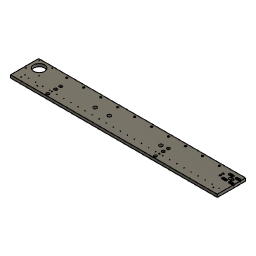
XPlate v29 (Autodesk Fusion 360 archive; units mm, degrees)
design "XPlate" references "tormach 770mx"
Autodesk Fusion 360 part; units mm, degrees
sketch "Sketch1" plane through (0, 0, 0) normal (0, 1, 0) x (1, 0, 0)
  line L0 (0, 0) -> (732, 0)
  line L1 (732, 0) -> (732, -100)
  line L2 (732, -100) -> (0, -100)
  line L3 (0, -100) -> (0, 0)
  dimension "d1" = 732
  dimension "d2" = 100
  constraint horizontal L0
  constraint vertical L1
  constraint horizontal L2
  constraint vertical L3
  constraint coincident L0.start L3.end
  measures "d1" distance of L0.start L0.end
  measures "d2" distance of L0.start L2.end
extrude "Extrude1" add sketch "Sketch1" along normal blind 9.6
sketch "Sketch2" plane through (0, 9.6, 0) normal (0, 1, 0) x (-1, 0, 0)
  line L0 (0, 100) -> (-732, 100)
  line L1 (-732, 100) -> (-732, 0)
  line L2 (-732, 0) -> (0, 0)
  line L3 (0, 0) -> (0, 100)
  line L4 (0, 28.5) -> (-732, 28.5) construction
  line L5 (-707, 23.5) -> (-713, 23.5)
  line L6 (-707, 33.5) -> (-712.9996, 33.5)
  arc A0 (-707, 23.5) -> (-707, 33.5) centre (-707, 28.5) ccw
  arc A1 (-712.9996, 33.5) -> (-713, 23.5) centre (-713, 28.5) ccw
  line L7 (0, 16.5) -> (-732, 16.5) construction
  line L8 (-693, 20.5) -> (-703, 20.5)
  arc A2 (-703, 20.5) -> (-703, 12.5) centre (-703, 16.5) ccw
  line L9 (-703, 12.5) -> (-693, 12.5)
  arc A3 (-693, 12.5) -> (-693, 20.5) centre (-693, 16.5) ccw
  line L10 (-693, 16.5) -> (-703, 16.5) construction
  line L11 (-717, 20.5) -> (-727, 20.5)
  arc A4 (-727, 20.5) -> (-727, 12.5) centre (-727, 16.5) ccw
  line L12 (-727, 12.5) -> (-717, 12.5)
  arc A5 (-717, 12.5) -> (-717, 20.5) centre (-717, 16.5) ccw
  line L13 (-717, 16.5) -> (-727, 16.5) construction
  line L14 (-694.5, 18.75) -> (-701.5, 18.75)
  arc A6 (-701.5, 18.75) -> (-701.5, 14.25) centre (-701.5, 16.5) ccw
  line L15 (-701.5, 14.25) -> (-694.5, 14.25)
  arc A7 (-694.5, 14.25) -> (-694.5, 18.75) centre (-694.5, 16.5) ccw
  line L16 (-694.5, 16.5) -> (-701.5, 16.5) construction
  line L17 (-718.5, 18.75) -> (-725.5, 18.75)
  arc A8 (-725.5, 18.75) -> (-725.5, 14.25) centre (-725.5, 16.5) ccw
  line L18 (-725.5, 14.25) -> (-718.5, 14.25)
  arc A9 (-718.5, 14.25) -> (-718.5, 18.75) centre (-718.5, 16.5) ccw
  line L19 (-718.5, 16.5) -> (-725.5, 16.5) construction
  line L20 (-693, 16.5) -> (-693, 44) construction
  line L21 (-694.5, 16.5) -> (-694.5, 18.75) construction
  line L22 (-703, 16.5) -> (-703, 44) construction
  line L23 (-694.5, 16.5) -> (-694.5, 44) construction
  line L24 (-701.5, 16.5) -> (-701.5, 44) construction
  line L25 (-717, 16.5) -> (-717, 44) construction
  line L26 (-718.5, 16.5) -> (-718.5, 44) construction
  line L27 (-725.5, 16.5) -> (-725.5, 44) construction
  line L28 (-727, 16.5) -> (-727, 44) construction
  line L29 (-689, 40.5) -> (-732, 40.5) construction
  line L30 (-694.5, 42.75) -> (-701.5, 42.75)
  arc A10 (-701.5, 42.75) -> (-701.5, 38.25) centre (-701.5, 40.5) ccw
  line L31 (-701.5, 38.25) -> (-694.5, 38.25)
  arc A11 (-694.5, 38.25) -> (-694.5, 42.75) centre (-694.5, 40.5) ccw
  line L32 (-694.5, 40.5) -> (-701.5, 40.5) construction
  line L33 (-693, 44.5) -> (-703, 44.5)
  arc A12 (-703, 44.5) -> (-703, 36.5) centre (-703, 40.5) ccw
  line L34 (-703, 36.5) -> (-693, 36.5)
  arc A13 (-693, 36.5) -> (-693, 44.5) centre (-693, 40.5) ccw
  line L35 (-693, 40.5) -> (-703, 40.5) construction
  line L36 (-718.5, 42.75) -> (-725.5, 42.75)
  arc A14 (-725.5, 42.75) -> (-725.5, 38.25) centre (-725.5, 40.5) ccw
  line L37 (-725.5, 38.25) -> (-718.5, 38.25)
  arc A15 (-718.5, 38.25) -> (-718.5, 42.75) centre (-718.5, 40.5) ccw
  line L38 (-718.5, 40.5) -> (-725.5, 40.5) construction
  line L39 (-717, 44.5) -> (-727, 44.5)
  arc A16 (-727, 44.5) -> (-727, 36.5) centre (-727, 40.5) ccw
  line L40 (-727, 36.5) -> (-717, 36.5)
  arc A17 (-717, 36.5) -> (-717, 44.5) centre (-717, 40.5) ccw
  line L41 (-717, 40.5) -> (-727, 40.5) construction
  line L42 (0, 8.9342) -> (-760, 8.9342) construction
  line L43 (0, 78) -> (-732, 78) construction
  line L44 (-124, 46) -> (-124, 92) construction
  line L45 (-505, 46) -> (-505, 92) construction
  line L46 (0, 86) -> (-732, 86) construction
  line L47 (-30, 0) -> (-30, 60) construction
  line L48 (-53.57, 4.93) -> (-6.43, 4.93) construction
  line L49 (-6.43, 4.93) -> (-6.43, 52.07) construction
  line L50 (-6.43, 52.07) -> (-53.57, 52.07) construction
  line L51 (-53.57, 52.07) -> (-53.57, 4.93) construction
  line L52 (-53.57, 4.93) -> (-6.43, 52.07) construction
  line L53 (-6.43, 4.93) -> (-53.57, 52.07) construction
  circle A18 centre (-30, 28.5) radius 19.75
  line L54 (-250, 0) -> (-250, 100) construction
  line L55 (-482, 0) -> (-482, 100) construction
  line L56 (-250, 50) -> (-482, 50) construction
  line L57 (-300, 0) -> (-300, 100) construction
  point P0 (-713, 28.5)
  point P1 (-707, 28.5)
  point P2 (-693, 16.5)
  point P3 (-703, 16.5)
  point P4 (-693, 16.5)
  point P5 (-717, 16.5)
  point P6 (-727, 16.5)
  point P7 (-694.5, 16.5)
  point P8 (-701.5, 16.5)
  point P9 (-718.5, 16.5)
  point P10 (-725.5, 16.5)
  point P11 (-693, 40.5)
  point P12 (-694.5, 40.5)
  point P13 (-701.5, 40.5)
  point P14 (-703, 40.5)
  point P15 (-717, 40.5)
  point P16 (-718.5, 40.5)
  point P17 (-725.5, 40.5)
  point P18 (-727, 40.5)
  point P19 (-678.99, 26.59)
  point P20 (-678.99, 36.59)
  point P21 (-124, 46)
  point P22 (-124, 64)
  point P23 (-124, 92)
  point P24 (-505, 46)
  point P25 (-505, 64)
  point P26 (-505, 92)
  point P27 (-108.4571, 8.9342)
  point P28 (-25.5, 74)
  point P29 (-25.5, 87.18)
  point P30 (-717, 78)
  point P31 (-505, 78)
  point P32 (-124, 78)
  point P33 (-80.74, 86)
  point P34 (-30, 28.5)
  point P35 (-53.57, 4.93)
  point P36 (-6.43, 4.93)
  point P37 (-6.43, 52.07)
  point P38 (-53.57, 52.07)
  point P39 (-250, 50)
  point P40 (-482, 50)
  point P41 (-300, 50)
  dimension "d5" = 28.5
  dimension "d6" = 19
  dimension "d7" = 6
  dimension "d8" = 10
  dimension "d9" = 10
  dimension "d11" = 16.5
  dimension "d12" = 10
  dimension "d13" = 29
  dimension "d19" = 8
  dimension "d20" = 10
  dimension "d21" = 5
  dimension "d22" = 8
  dimension "d23" = 7
  dimension "d24" = 7
  dimension "d25" = 30.5
  dimension "d26" = 4.5
  dimension "d27" = 6.5
  dimension "d28" = 4.5
  dimension "d29" = 40.5
  dimension "d30" = 4.5
  dimension "d31" = 8
  dimension "d32" = 4.5
  dimension "d33" = 8
  dimension "d37" = 10
  dimension "d38" = 53.01
  dimension "d39" = 26.59
  dimension "d50" = 381
  dimension "d51" = 28
  dimension "d52" = 18
  dimension "d53" = 8
  dimension "d54" = 124
  dimension "d74" = 8.9342
  dimension "d75" = 108.4571
  dimension "d85" = 13.18
  dimension "d86" = 25.5
  dimension "d93" = 22
  dimension "d94" = 15
  dimension "d112" = 14
  dimension "d113" = 80.74
  dimension "d121" = 30
  dimension "d123" = 47.14
  dimension "d124" = 47.14
  dimension "d137" = 39.5
  dimension "d139" = 12.82
  dimension "d140" = 250
  dimension "d141" = 250
  dimension "d152" = 300
  constraint coincident L3 L4.start
  constraint coincident L1 L4.end
  constraint perpendicular L1 L4
  constraint coincident L4 P0
  constraint coincident L4 P1
  constraint coincident P1 A0.centre
  constraint coincident P0 A1.centre
  constraint tangent L5 A1
  constraint tangent L6 A0
  constraint parallel L5 L6
  constraint coincident L3 L7.start
  constraint coincident L1 L7.end
  constraint perpendicular L1 L7
  constraint coincident L7 P4
  constraint coincident L7 P3
  constraint tangent L5 A0
  constraint tangent L8 A2
  constraint tangent A2 L9
  constraint parallel L8 L9
  constraint tangent L9 A3
  constraint tangent L8 A3
  constraint coincident P3 A2.centre
  constraint parallel L7 L10
  constraint coincident P4 P2
  constraint coincident L7 P5
  constraint coincident L7 P6
  constraint tangent L11 A4
  constraint tangent A4 L12
  constraint parallel L11 L12
  constraint tangent L12 A5
  constraint tangent L11 A5
  constraint coincident P6 A4.centre
  constraint parallel L7 L13
  constraint coincident P5 A5.centre
  constraint coincident L7 P7
  constraint coincident L7 P8
  constraint coincident L13 P9
  constraint coincident L13 P10
  constraint tangent L14 A6
  constraint tangent A6 L15
  constraint parallel L14 L15
  constraint tangent L15 A7
  constraint tangent L14 A7
  constraint coincident P8 A6.centre
  constraint parallel L7 L16
  constraint coincident P7 A7.centre
  constraint tangent L17 A8
  constraint tangent A8 L18
  constraint parallel L17 L18
  constraint tangent L18 A9
  constraint tangent L17 A9
  constraint coincident P10 A8.centre
  constraint parallel L7 L19
  constraint coincident P9 A9.centre
  constraint perpendicular L4 L20
  constraint perpendicular L4 L22
  constraint perpendicular L4 L23
  constraint perpendicular L4 L24
  constraint perpendicular L4 L25
  constraint perpendicular L4 L26
  constraint perpendicular L4 L27
  constraint perpendicular L4 L28
  constraint coincident L1 L29.end
  constraint perpendicular L1 L29
  constraint coincident L29 P11
  constraint coincident L20 P11
  constraint coincident L29 P12
  constraint coincident L23 P12
  constraint coincident L24 P13
  constraint coincident L29 P13
  constraint coincident L29 P14
  constraint coincident L22 P14
  constraint coincident L25 P15
  constraint coincident L29 P15
  constraint coincident L26 P16
  constraint coincident L29 P16
  constraint coincident L27 P17
  constraint coincident L29 P17
  constraint coincident L29 P18
  constraint coincident L28 P18
  constraint tangent L30 A10
  constraint tangent A10 L31
  constraint parallel L30 L31
  constraint tangent L31 A11
  constraint tangent L30 A11
  constraint coincident P13 A10.centre
  constraint perpendicular L24 L32
  constraint coincident P12 A11.centre
  constraint tangent L33 A12
  constraint tangent A12 L34
  constraint parallel L33 L34
  constraint tangent L34 A13
  constraint tangent L33 A13
  constraint coincident P14 A12.centre
  constraint perpendicular L22 L35
  constraint coincident P11 A13.centre
  constraint tangent L36 A14
  constraint tangent A14 L37
  constraint parallel L36 L37
  constraint tangent L37 A15
  constraint tangent L36 A15
  constraint coincident P17 A14.centre
  constraint perpendicular L27 L38
  constraint coincident P16 A15.centre
  constraint tangent L39 A16
  constraint tangent A16 L40
  constraint parallel L39 L40
  constraint tangent L40 A17
  constraint tangent L39 A17
  constraint coincident P18 A16.centre
  constraint perpendicular L28 L41
  constraint coincident P15 A17.centre
  constraint vertical P19 P20
  constraint vertical P21 P22
  constraint vertical P22 P23
  constraint vertical P24 P25
  constraint vertical P25 P26
  constraint horizontal P23 P26
  constraint horizontal P22 P25
  constraint horizontal P21 P24
  constraint coincident L3 L42.start
  constraint perpendicular L1 L42
  constraint coincident L42 P27
  constraint vertical P28 P29
  constraint coincident L3 L43.start
  constraint coincident L1 L43.end
  constraint perpendicular L1 L43
  constraint coincident L43 P30
  constraint coincident P21 L44.start
  constraint coincident P23 L44.end
  constraint coincident P24 L45.start
  constraint coincident P26 L45.end
  constraint coincident L45 P31
  constraint coincident L43 P31
  constraint coincident L43 P32
  constraint coincident L44 P32
  constraint coincident L3 L46.start
  constraint coincident L1 L46.end
  constraint perpendicular L1 L46
  constraint coincident L46 P33
  constraint coincident L2 L47.start
  constraint perpendicular L4 L47
  constraint horizontal L48
  constraint perpendicular L48 L49
  constraint parallel L48 L50
  constraint parallel L49 L51
  constraint coincident L52 P34
  constraint coincident L53 P34
  constraint coincident L4 P34
  constraint coincident L47 P34
  constraint coincident P35 L48.start
  constraint coincident P36 L48.end
  constraint coincident P37 L49.end
  constraint coincident P38 L50.end
  constraint coincident P34 A18.centre
  constraint coincident L2 L54.start
  constraint coincident L0 L54.end
  constraint perpendicular L0 L54
  constraint coincident L2 L55.start
  constraint coincident L0 L55.end
  constraint perpendicular L0 L55
  constraint midpoint L54 P39
  constraint midpoint L55 P40
  constraint coincident P39 L56.start
  constraint coincident P40 L56.end
  constraint coincident L2 L57.start
  constraint coincident L0 L57.end
  constraint perpendicular L0 L57
  constraint midpoint L57 P41
  measures "d5" distance of L2 L4
  measures "d6" distance of L1 P0
  measures "d7" distance of P0 P1
  measures "d8" diameter of A0
  measures "d9" diameter of A1
  measures "d11" distance of L2 L7
  measures "d12" distance of P4 P3
  measures "d13" distance of L1 P3
  measures "d19" diameter of A2
  measures "d20" distance of P5 P6
  measures "d21" distance of L1 P6
  measures "d22" diameter of A4
  measures "d23" distance of P7 P8
  measures "d24" distance of P9 P10
  measures "d25" distance of L1 P8
  measures "d26" diameter of A6
  measures "d27" distance of L1 P10
  measures "d28" diameter of A8
  measures "d29" distance of L2 L29
  measures "d30" diameter of A10
  measures "d31" diameter of A12
  measures "d32" diameter of A14
  measures "d33" diameter of A16
  measures "d37" distance of P19 P20
  measures "d38" distance of L1 P20
  measures "d39" distance of L2 P19
  measures "d50" distance of P23 P26
  measures "d51" distance of P22 P23
  measures "d52" distance of P21 P22
  measures "d53" distance of L0 P23
  measures "d54" distance of L3 P23
  measures "d74" distance of L2 L42
  measures "d75" distance of L3 P27
  measures "d85" distance of P28 P29
  measures "d86" distance of L3 P29
  measures "d93" distance of L0 L43
  measures "d94" distance of L1 P30
  measures "d112" distance of L0 L46
  measures "d113" distance of L3 P33
  measures "d121" distance of L3 L47
  measures "d123" distance of P37 P38
  measures "d124" distance of P36 P37
  measures "d137" diameter of A18
  measures "d139" distance of L0 P29
  measures "d140" distance of L3 L54
  measures "d141" distance of L1 L55
  measures "d152" distance of L3 L57
extrude "Extrude2" cut sketch "Sketch2" along normal through all and the other way through all contours L5 L6 A0 A1
extrude "Extrude3" cut sketch "Sketch2" along normal through all and the other way through all contours L14 A6 L15 A7 | L17 A8 L18 A9 | L30 A10 L31 A11 | L36 A14 L37 A15
extrude "Extrude4" cut sketch "Sketch2" against normal blind 4 contours L8 A2 L9 A3 | L11 A4 L12 A5 | L33 A12 L34 A13 | L39 A16 L40 A17
hole "Hole1" at (678.99, 9.6, 26.59) direction (0, -1, 0) diameter 3.4 end through all counterbore diameter 6.5 counterbore depth 3
hole "Hole2" at (678.99, 9.6, 36.59) direction (0, -1, 0) diameter 3.4 end through all counterbore diameter 6.5 counterbore depth 3
hole "Hole3" at (124, 9.6, 46) direction (0, -1, 0) diameter 5.3 end through all counterbore diameter 10.1 counterbore depth 5
hole "Hole4" at (124, 9.6, 64) direction (0, -1, 0) diameter 5.3 end through all counterbore diameter 10.1 counterbore depth 5
hole "Hole5" at (124, 9.6, 92) direction (0, -1, 0) diameter 5.3 end through all counterbore diameter 10.1 counterbore depth 5
pattern_linear "R-Pattern1" count 1 spacing 0 along (0, 0, -1) count 2 spacing 381 along (1, 0, 0) of "Hole3", "Hole4", "Hole5"
hole "Hole6" at (108.4571, 9.6, 8.9342) direction (0, -1, 0) diameter 3.4 end through all counterbore diameter 6.5 counterbore depth 3
pattern_linear "R-Pattern2" count 1 spacing 0 along (0, 0, 1) count 10 spacing 60 along (1, 0, 0) of "Hole6"
hole "Hole7" at (25.5, 9.6, 74) direction (0, -1, 0) diameter 2.5 end through all
hole "Hole8" at (25.5, 9.6, 87.18) direction (0, -1, 0) diameter 3 end through all
hole "Hole9" at (717, 9.6, 78) direction (0, -1, 0) diameter 2.5 end through all
pattern_linear "R-Pattern3" count 1 spacing 0 along (0, 0, -1) count 28 spacing 25 along (-1, 0, 0) of "Hole9"
hole "Hole11" at (124, 9.6, 78) direction (0, -1, 0) diameter 3.9 depth 10 tip angle 118
pattern_linear "R-Pattern4" count 1 spacing 0 along (0, 0, -1) count 2 spacing 381 along (1, 0, 0) of "Hole11"
hole "Hole12" at (80.74, 9.6, 86) direction (0, -1, 0) diameter 3.8 end through all
pattern_linear "R-Pattern5" count 1 spacing 0 along (0, 0, -1) count 2 spacing 623.5772 along (1, 0, 0) of "Hole12"
hole "Hole13" at (6.43, 9.6, 4.93) direction (0, -1, 0) diameter 3.3 end through all
hole "Hole14" at (53.57, 9.6, 4.93) direction (0, -1, 0) diameter 3.3 end through all
hole "Hole15" at (53.57, 9.6, 52.07) direction (0, -1, 0) diameter 3.3 end through all
hole "Hole16" at (6.43, 9.6, 52.07) direction (0, -1, 0) diameter 3.3 end through all
extrude "Extrude5" cut sketch "Sketch2" along normal through all and the other way through all contours A18
hole "Hole17" at (250, 9.6, 50) direction (0, -1, 0) diameter 12 end through all
hole "Hole19" at (482, 9.6, 50) direction (0, -1, 0) diameter 12 depth 10 tip angle 118
hole "Hole20" at (300, 9.6, 50) direction (0, -1, 0) diameter 12 depth 80 tip angle 118
